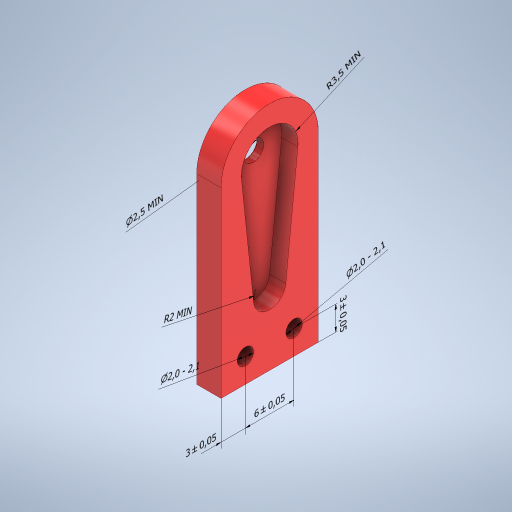
# Autodesk Inventor part: rapoukMiddleLeg2v3
Saved by Autodesk Inventor 2024 (Build 280153000, 153)
## iProperties
Created: 2023-05-29
Part Number: rapoukMiddleLeg2v3
Material: EN AW-6060 T6
Document SubType Name: Modeling
Designer: Roman
Density: 2.7 g/cm^3
Appearance: Light Red
Description: Hybná část nohy
Mass: 1.98295 g
Surface Area: 9.92124 cm^2
Volume: 0.734426 cm^3
Polotovar: KR...
Author: Roman
## iProperties of the stored document middleLegv2-2_3DPrint.ipt
Created: 2023-06-18
Part Number: middleLegv2-2_3DPrint
Material: Generic
Document SubType Name: Modeling
Designer: Roman
Density: 1 g/cm^3
Appearance: Default
Author: Roman
Autodesk Inventor part; units mm, degrees
ref_plane "YZ Plane" through (0, 0, 0) normal (1, 0, 0) x (0, 1, 0)
ref_plane "XZ Plane" through (0, 0, 0) normal (0, 1, 0) x (-1, 0, 0)
ref_plane "XY Plane" through (0, 0, 0) normal (0, 0, 1) x (1, 0, 0)
sketch "Sketch1" plane through (0, 0, 0) normal (0, 1, 0) x (-1, 0, 0)
  line L0 (-1.5, 6) -> (1.5, 6)
  line L1 (1.5, 6) -> (1.5, -6)
  line L2 (1.5, -6) -> (-1.5, -6)
  line L3 (-1.5, -6) -> (-1.5, 6)
  line L4 (-1.5, 6) -> (1.5, -6) construction
  line L5 (1.5, 6) -> (-1.5, -6) construction
  point P0 (0, 0)
  dimension "d0" = 3
  dimension "d1" = 12
  constraints: 12 end point, 2 midpoint, 2 parallel, 1 horizontal, 1 perpendicular
  measures "d0" distance of L1.end L2.end
  measures "d1" distance of L0.end L1.end
extrude "Extrusion1" add sketch "Sketch1" along normal blind 28.5
fillet "Fillet1" radius 6 2 edges at (0, 28.5, 6) (0, 28.5, -6)
sketch "Sketch3" plane through (1.5, 0, 6) normal (1, 0, 0) x (0, 0, -1)
  arc A0 (12, 22.5) -> (0, 22.5) centre (6, 22.5) ccw projected
  arc A1 (9.4799, 22.125) -> (2.5201, 22.125) centre (6, 22.5) ccw
  line L0 (6, 22.5) -> (6, 8.5) construction
  line L1 (6, 22.5) -> (20, 22.5) construction
  arc A2 (4.0115, 8.2857) -> (7.9885, 8.2857) centre (6, 8.5) ccw
  line L2 (4.0115, 8.2857) -> (2.5201, 22.125)
  line L3 (7.9885, 8.2857) -> (9.4799, 22.125)
  circle A3 centre (6, 22.5) radius 1.25
  point P0 (6, 0)
  dimension "d8" = 7
  dimension "d9" = 14
  dimension "d10" = 90
  dimension "d11" = 4
  dimension "d43" = 2.5
  constraints: 8 end point, 4 point on circle, 4 tangent, 3 centre point, 3 coincident, 1 horizontal, 1 perpendicular, 1 vertical
  measures "d8" diameter of A1
  measures "d9" distance of L0.start L0.end
  measures "d10" angle of L0 L1
  measures "d11" diameter of A2
  measures "d43" diameter of A3
extrude "Extrusion3" cut sketch "Sketch3" against normal blind 2
sketch "Sketch6" plane through (-1.5, 0, -6) normal (-1, 0, 0) x (0, 0, 1)
  line L0 (6, 0) -> (6, 28.5)
  arc A0 (12, 22.5) -> (0, 22.5) centre (6, 22.5) ccw projected
  line L1 (0, 0) -> (12, 0) construction
  line L2 (0, 0) -> (3, 0) construction
  line L3 (3, 0) -> (3, 3) construction
  line L4 (3, 3) -> (0, 3) construction
  line L5 (0, 3) -> (0, 0) construction
  line L6 (9, 0) -> (9, 3) construction
  line L7 (9, 3) -> (12, 3) construction
  dimension "d35" = 3
  constraints: 14 end point, 3 symmetric about line, 2 parallel, 2 perpendicular, 1 horizontal, 1 point on circle, 1 vertical
  measures "d35" distance of L4.end L3.end
hole "Hole2" at (-1.5, 3, -3) at (-1.5, 3, 3) direction (1, 0, 0) diameter 2 depth 3 countersink diameter 2.5 countersink angle 90
extrude "Vysunutí6" cut sketch "Sketch3" against normal through all contours A3
chamfer "Chamfer1" distance 0.2 angle 45 1 edges at (-1.5, 22.5, 1.25)
body "Solid1"
